Autodesk Fusion 360 part; units mm, degrees
note: some values were not read from the file. Chosen so that the rebuilt part matches the saved one: which bodies a step acts on. Set by a fixed rule: which sketch regions a step uses.
(part 3 of 5)
extrude "Extrude1'''" add sketch "Sketch1 (2)" along normal blind 15 separate body contours L572 L573 L574 L575 picked at (-36.083333, 0.25) makes body 9 in component "grid_3d"
sketch "Sketch2 (3)" plane through (0, 0, -3) normal (0, 0, 1) x (-1, 0, 0) in component "grid_3d"
  line L0 (-108.25, 0.75) -> (-108.25, -0.75)
  line L1 (-108.25, -0.75) -> (108.25, -0.75)
  line L2 (108.25, -0.75) -> (108.25, 0.75)
  line L3 (108.25, 0.75) -> (-108.25, 0.75)
  arc A0 (86, 102) -> (87, 101) centre (87, 102) ccw
  line L4 (87, 101) -> (100.585786, 101)
  arc A1 (100.585786, 101) -> (101.292893, 101.292893) centre (100.585786, 102) ccw
  line L5 (101.292893, 101.292893) -> (116.946699, 116.946699)
  arc A2 (116.946699, 116.946699) -> (122.25, 129.75) centre (122.25, 122.25) ccw
  line L6 (122.25, 129.75) -> (-116.02505, 129.75)
  arc A3 (-116.02505, 129.75) -> (-116.716711, 128.027778) centre (-116.02505, 128.75) ccw
  arc A4 (-115.999634, 117.256712) -> (-116.716711, 128.027778) centre (-122.25, 122.25) ccw
  arc A5 (-115.999634, 117.256712) -> (-115.925445, 115.925445) centre (-115.218338, 116.632551) ccw
  line L7 (-115.925445, 115.925445) -> (-101.292893, 101.292893)
  arc A6 (-101.292893, 101.292893) -> (-100.585786, 101) centre (-100.585786, 102) ccw
  line L8 (-100.585786, 101) -> (-87, 101)
  arc A7 (-87, 101) -> (-86, 102) centre (-87, 102) ccw
  line L9 (-86, 102) -> (-86, 108.5)
  line L10 (-86, 108.5) -> (-84, 108.5)
  line L11 (-84, 108.5) -> (-84, 102)
  arc A8 (-84, 102) -> (-83, 101) centre (-83, 102) ccw
  line L12 (-83, 101) -> (-70, 101)
  arc A9 (-70, 101) -> (-69, 102) centre (-70, 102) ccw
  line L13 (-69, 102) -> (-69, 108.5)
  line L14 (-69, 108.5) -> (-67, 108.5)
  line L15 (-67, 108.5) -> (-67, 102)
  arc A10 (-67, 102) -> (-66, 101) centre (-66, 102) ccw
  line L16 (-66, 101) -> (-53, 101)
  arc A11 (-53, 101) -> (-52, 102) centre (-53, 102) ccw
  line L17 (-52, 102) -> (-52, 108.5)
  line L18 (-52, 108.5) -> (-50, 108.5)
  line L19 (-50, 108.5) -> (-50, 102)
  arc A12 (-50, 102) -> (-49, 101) centre (-49, 102) ccw
  line L20 (-49, 101) -> (-36, 101)
  arc A13 (-36, 101) -> (-35, 102) centre (-36, 102) ccw
  line L21 (-35, 102) -> (-35, 108.5)
  line L22 (-35, 108.5) -> (-33, 108.5)
  line L23 (-33, 108.5) -> (-33, 102)
  arc A14 (-33, 102) -> (-32, 101) centre (-32, 102) ccw
  line L24 (-32, 101) -> (-19, 101)
  arc A15 (-19, 101) -> (-18, 102) centre (-19, 102) ccw
  line L25 (-18, 102) -> (-18, 108.5)
  line L26 (-18, 108.5) -> (-16, 108.5)
  line L27 (-16, 108.5) -> (-16, 102)
  arc A16 (-16, 102) -> (-15, 101) centre (-15, 102) ccw
  line L28 (-15, 101) -> (-2, 101)
  arc A17 (-2, 101) -> (-1, 102) centre (-2, 102) ccw
  line L29 (-1, 102) -> (-1, 108.5)
  line L30 (-1, 108.5) -> (1, 108.5)
  line L31 (1, 108.5) -> (1, 102)
  arc A18 (1, 102) -> (2, 101) centre (2, 102) ccw
  line L32 (2, 101) -> (15, 101)
  arc A19 (15, 101) -> (16, 102) centre (15, 102) ccw
  line L33 (16, 102) -> (16, 108.5)
  line L34 (16, 108.5) -> (18, 108.5)
  line L35 (18, 108.5) -> (18, 102)
  arc A20 (18, 102) -> (19, 101) centre (19, 102) ccw
  line L36 (19, 101) -> (32, 101)
  arc A21 (32, 101) -> (33, 102) centre (32, 102) ccw
  line L37 (33, 102) -> (33, 108.5)
  line L38 (33, 108.5) -> (35, 108.5)
  line L39 (35, 108.5) -> (35, 102)
  arc A22 (35, 102) -> (36, 101) centre (36, 102) ccw
  line L40 (36, 101) -> (49, 101)
  arc A23 (49, 101) -> (50, 102) centre (49, 102) ccw
  line L41 (50, 102) -> (50, 108.5)
  line L42 (50, 108.5) -> (52, 108.5)
  line L43 (52, 108.5) -> (52, 102)
  arc A24 (52, 102) -> (53, 101) centre (53, 102) ccw
  line L44 (53, 101) -> (66, 101)
  arc A25 (66, 101) -> (67, 102) centre (66, 102) ccw
  line L45 (67, 102) -> (67, 108.5)
  line L46 (67, 108.5) -> (69, 108.5)
  line L47 (69, 108.5) -> (69, 102)
  arc A26 (69, 102) -> (70, 101) centre (70, 102) ccw
  line L48 (70, 101) -> (83, 101)
  arc A27 (83, 101) -> (84, 102) centre (83, 102) ccw
  line L49 (84, 102) -> (84, 108.5)
  line L50 (84, 108.5) -> (86, 108.5)
  line L51 (86, 108.5) -> (86, 102)
  circle A28 centre (-17, 118.5) radius 7.5
  circle A29 centre (34, 118.5) radius 7.5
  circle A30 centre (17, 118.5) radius 7.5
  circle A31 centre (122.25, 122.25) radius 2.5
  circle A32 centre (-34, 118.5) radius 7.5
  circle A33 centre (0, 118.5) radius 7.5
  arc A34 (-86, -102) -> (-87, -101) centre (-87, -102) ccw
  line L52 (-87, -101) -> (-100.585786, -101)
  arc A35 (-100.585786, -101) -> (-101.292893, -101.292893) centre (-100.585786, -102) ccw
  line L53 (-101.292893, -101.292893) -> (-116.946699, -116.946699)
  arc A36 (-116.946699, -116.946699) -> (-122.25, -129.75) centre (-122.25, -122.25) ccw
  line L54 (-122.25, -129.75) -> (116.02505, -129.75)
  arc A37 (116.02505, -129.75) -> (116.716711, -128.027778) centre (116.02505, -128.75) ccw
  arc A38 (115.999634, -117.256712) -> (116.716711, -128.027778) centre (122.25, -122.25) ccw
  arc A39 (115.999634, -117.256712) -> (115.925445, -115.925445) centre (115.218338, -116.632551) ccw
  line L55 (115.925445, -115.925445) -> (101.292893, -101.292893)
  arc A40 (101.292893, -101.292893) -> (100.585786, -101) centre (100.585786, -102) ccw
  line L56 (100.585786, -101) -> (87, -101)
  arc A41 (87, -101) -> (86, -102) centre (87, -102) ccw
  line L57 (86, -102) -> (86, -108.5)
  line L58 (86, -108.5) -> (84, -108.5)
  line L59 (84, -108.5) -> (84, -102)
  arc A42 (84, -102) -> (83, -101) centre (83, -102) ccw
  line L60 (83, -101) -> (70, -101)
  arc A43 (70, -101) -> (69, -102) centre (70, -102) ccw
  line L61 (69, -102) -> (69, -108.5)
  line L62 (69, -108.5) -> (67, -108.5)
  line L63 (67, -108.5) -> (67, -102)
  arc A44 (67, -102) -> (66, -101) centre (66, -102) ccw
  line L64 (66, -101) -> (53, -101)
  arc A45 (53, -101) -> (52, -102) centre (53, -102) ccw
  line L65 (52, -102) -> (52, -108.5)
  line L66 (52, -108.5) -> (50, -108.5)
  line L67 (50, -108.5) -> (50, -102)
  arc A46 (50, -102) -> (49, -101) centre (49, -102) ccw
  line L68 (49, -101) -> (36, -101)
  arc A47 (36, -101) -> (35, -102) centre (36, -102) ccw
  line L69 (35, -102) -> (35, -108.5)
  line L70 (35, -108.5) -> (33, -108.5)
  line L71 (33, -108.5) -> (33, -102)
  arc A48 (33, -102) -> (32, -101) centre (32, -102) ccw
  line L72 (32, -101) -> (19, -101)
  arc A49 (19, -101) -> (18, -102) centre (19, -102) ccw
  line L73 (18, -102) -> (18, -108.5)
  line L74 (18, -108.5) -> (16, -108.5)
  line L75 (16, -108.5) -> (16, -102)
  arc A50 (16, -102) -> (15, -101) centre (15, -102) ccw
  line L76 (15, -101) -> (2, -101)
  arc A51 (2, -101) -> (1, -102) centre (2, -102) ccw
  line L77 (1, -102) -> (1, -108.5)
  line L78 (1, -108.5) -> (-1, -108.5)
  line L79 (-1, -108.5) -> (-1, -102)
  arc A52 (-1, -102) -> (-2, -101) centre (-2, -102) ccw
  line L80 (-2, -101) -> (-15, -101)
  arc A53 (-15, -101) -> (-16, -102) centre (-15, -102) ccw
  line L81 (-16, -102) -> (-16, -108.5)
  line L82 (-16, -108.5) -> (-18, -108.5)
  line L83 (-18, -108.5) -> (-18, -102)
  arc A54 (-18, -102) -> (-19, -101) centre (-19, -102) ccw
  line L84 (-19, -101) -> (-32, -101)
  arc A55 (-32, -101) -> (-33, -102) centre (-32, -102) ccw
  line L85 (-33, -102) -> (-33, -108.5)
  line L86 (-33, -108.5) -> (-35, -108.5)
  line L87 (-35, -108.5) -> (-35, -102)
  arc A56 (-35, -102) -> (-36, -101) centre (-36, -102) ccw
  line L88 (-36, -101) -> (-49, -101)
  arc A57 (-49, -101) -> (-50, -102) centre (-49, -102) ccw
  line L89 (-50, -102) -> (-50, -108.5)
  line L90 (-50, -108.5) -> (-52, -108.5)
  line L91 (-52, -108.5) -> (-52, -102)
  arc A58 (-52, -102) -> (-53, -101) centre (-53, -102) ccw
  line L92 (-53, -101) -> (-66, -101)
  arc A59 (-66, -101) -> (-67, -102) centre (-66, -102) ccw
  line L93 (-67, -102) -> (-67, -108.5)
  line L94 (-67, -108.5) -> (-69, -108.5)
  line L95 (-69, -108.5) -> (-69, -102)
  arc A60 (-69, -102) -> (-70, -101) centre (-70, -102) ccw
  line L96 (-70, -101) -> (-83, -101)
  arc A61 (-83, -101) -> (-84, -102) centre (-83, -102) ccw
  line L97 (-84, -102) -> (-84, -108.5)
  line L98 (-84, -108.5) -> (-86, -108.5)
  line L99 (-86, -108.5) -> (-86, -102)
  circle A62 centre (17, -118.5) radius 7.5
  circle A63 centre (-34, -118.5) radius 7.5
  circle A64 centre (-17, -118.5) radius 7.5
  circle A65 centre (-122.25, -122.25) radius 2.5
  circle A66 centre (34, -118.5) radius 7.5
  circle A67 centre (0, -118.5) radius 7.5
  line L100 (1, 129.75) -> (1, -129.75) construction
  line L101 (-1, 129.75) -> (-1, -129.75) construction
  line L102 (-1, 0.75) -> (1, 0.75)
  line L103 (1, 0.75) -> (1, -0.75)
  line L104 (1, -0.75) -> (-1, -0.75)
  line L105 (-1, -0.75) -> (-1, 0.75)
  line L106 (-86, -0.75) -> (-86, 0.75)
  line L107 (-84, 0.75) -> (-84, -0.75)
  line L108 (-69, -0.75) -> (-69, 0.75)
  line L109 (-67, 0.75) -> (-67, -0.75)
  line L110 (-52, -0.75) -> (-52, 0.75)
  line L111 (-50, 0.75) -> (-50, -0.75)
  line L112 (-35, -0.75) -> (-35, 0.75)
  line L113 (-33, 0.75) -> (-33, -0.75)
  line L114 (-18, -0.75) -> (-18, 0.75)
  line L115 (-16, 0.75) -> (-16, -0.75)
  line L116 (16, -0.75) -> (16, 0.75)
  line L117 (18, 0.75) -> (18, -0.75)
  line L118 (33, -0.75) -> (33, 0.75)
  line L119 (35, 0.75) -> (35, -0.75)
  line L120 (50, -0.75) -> (50, 0.75)
  line L121 (52, 0.75) -> (52, -0.75)
  line L122 (67, -0.75) -> (67, 0.75)
  line L123 (69, 0.75) -> (69, -0.75)
  line L124 (84, -0.75) -> (84, 0.75)
  line L125 (86, 0.75) -> (86, -0.75)
  line L126 (-85, 108.5) -> (-85, -108.5) construction
  dimension "d245" = 17
  dimension "d246" = 0
  constraint coincident L6 L100.start
  constraint coincident L54 L100.end
  constraint perpendicular L54 L100
  constraint coincident L6 L101.start
  constraint coincident L54 L101.end
  constraint perpendicular L54 L101
  constraint coincident A51.end L100
  constraint coincident L79.end L101
  constraint horizontal L102
  constraint vertical L103
  constraint horizontal L104
  constraint vertical L105
  constraint coincident L100 L103.end
  constraint coincident L1 L103.end
  constraint coincident L101 L102.start
  constraint coincident L3 L102.start
  constraint midpoint L10 L126.start
  constraint midpoint L98 L126.end
extrude "Extrude2'" cut sketch "Sketch2 (3)" against normal blind 7.75 contours L1 L3 L106 L107 | L1 L3 L108 L109 | L1 L3 L110 L111 | L1 L3 L112 L113 | L1 L3 L114 L115 | L1 L3 L102 L103 L104 L105 | L1 L3 L116 L117 | L1 L3 L118 L119 | L1 L3 L120 L121 | L1 L3 L122 L123 | L1 L3 L124 L125 picked at (-85.333333, 0.25) picked at (-68.333333, 0.25) picked at (-51.333333, 0.25) picked at (-34.333333, -0.25) picked at (-17.333333, -0.25) picked at (-0.333333, -0.25) picked at (16.666667, -0.25) picked at (33.666667, 0.25) picked at (50.666667, 0.25) picked at (67.666667, 0.25) picked at (84.666667, 0.25) bodies 9 in component "grid_3d"
pattern_linear "R-Pattern1" count 11 spacing 17 along (0, 1, 0) both ways of bodies 9 makes body 10 at (-100.833333, -85.75, -10.583333) makes body 11 at (-100.833333, -68.75, -10.583333) makes body 12 at (-100.833333, -51.75, -10.583333) makes body 13 at (-100.833333, -34.75, -10.583333) makes body 14 at (-100.833333, -17.75, -10.583333) makes body 15 at (-100.833333, 16.25, -10.583333) makes body 16 at (-100.833333, 33.25, -10.583333) makes body 17 at (-100.833333, 50.25, -10.583333) makes body 18 at (-100.833333, 67.25, -10.583333) makes body 19 at (-100.833333, 84.25, -10.583333) in component "grid_3d"
copy_body "CopyPasteBodies1" bodies 9 makes body 20 in component "grid_3d"
move_body "Move1" bodies 20 to x (0, 1, 0) y (1, 0, 0) z (0, 0, -1) at (0, 0, -21.5) in component "grid_3d"
extrude "Extrude3''" cut 12 faces at (-0.25, 100.833333, -18.5) (0.25, 79, -18.5) (-0.25, 57, -18.5) (-0.25, 40, -18.5) (-0.25, 28, -18.5) (0.25, 6, -18.5) (-0.25, -6, -18.5) (-0.25, -93.416667, -18.5) (-0.25, -74, -18.5) (-0.25, -57, -18.5) (-0.25, -40, -18.5) (-0.25, -23, -18.5) along direction (0, 0, 1) blind 1 on bodies 20 bodies 20 in component "grid_3d"
pattern_linear "R-Pattern2" count 11 spacing 17 along (1, 0, 0) both ways of bodies 20 makes body 21 at (-84.25, -100.833333, -10.583333) makes body 22 at (-67.25, -100.833333, -10.583333) makes body 23 at (-50.25, -100.833333, -10.583333) makes body 24 at (-33.25, -100.833333, -10.583333) makes body 25 at (-16.25, -100.833333, -10.583333) makes body 26 at (17.75, -100.833333, -10.583333) makes body 27 at (34.75, -100.833333, -10.583333) makes body 28 at (51.75, -100.833333, -10.583333) makes body 29 at (68.75, -100.833333, -10.583333) makes body 30 at (85.75, -100.833333, -10.583333) in component "grid_3d"
sketch "Sketch3 (3)" plane through (0, 0, -21) normal (0, 0, -1) x (1, 0, 0) in component "corner-bracket_3d"
  line L0 (110.5, 70.5) -> (105.75, 70.5)
  line L1 (105.75, 70.5) -> (105.75, 82.5)
  line L2 (105.75, 82.5) -> (110.5, 82.5)
  line L3 (110.5, 82.5) -> (110.5, 70.5)
  circle A0 centre (122.25, 61.125) radius 1.6
  line L4 (110.5, 87.5) -> (105.75, 87.5)
  line L5 (105.75, 87.5) -> (105.75, 99.5)
  line L6 (105.75, 99.5) -> (110.5, 99.5)
  line L7 (110.5, 99.5) -> (110.5, 87.5)
  line L8 (51, -124.5) -> (46.25, -124.5)
  line L9 (46.25, -124.5) -> (46.25, -112.5)
  line L10 (46.25, -112.5) -> (51, -112.5)
  line L11 (51, -112.5) -> (51, -124.5)
  circle A1 centre (0, 118.5) radius 7.5
  circle A2 centre (-61.125, -122.25) radius 1.6
  circle A3 centre (61.125, -122.25) radius 1.6
  circle A4 centre (122.25, -61.125) radius 1.6
  circle A5 centre (-61.125, 122.25) radius 1.6
  circle A6 centre (61.125, 122.25) radius 1.6
  circle A7 centre (-122.25, -61.125) radius 1.6
  circle A8 centre (-122.25, 61.125) radius 1.6
  circle A9 centre (-34, 123) radius 1.6
  circle A10 centre (-17, 123) radius 1.6
  circle A11 centre (17, 123) radius 1.6
  circle A12 centre (34, 123) radius 1.6
  circle A13 centre (-34, 114) radius 1.6
  circle A14 centre (17, 114) radius 1.6
  circle A15 centre (-17, 114) radius 1.6
  circle A16 centre (34, 114) radius 1.6
  circle A17 centre (-122.25, 122.25) radius 2.5
  circle A18 centre (-122.25, -122.25) radius 2.5
  line L12 (-105.75, -2.5) -> (-105.75, -14.5)
  line L13 (-105.75, -14.5) -> (-110.5, -14.5)
  line L14 (-110.5, -14.5) -> (-110.5, -2.5)
  line L15 (-110.5, -2.5) -> (-105.75, -2.5)
  line L16 (-105.75, -87.5) -> (-105.75, -99.5)
  line L17 (-105.75, -99.5) -> (-110.5, -99.5)
  line L18 (-110.5, -99.5) -> (-110.5, -87.5)
  line L19 (-110.5, -87.5) -> (-105.75, -87.5)
  circle A19 centre (122.25, 122.25) radius 2.5
  line L20 (-105.75, -19.5) -> (-105.75, -31.5)
  line L21 (-105.75, -31.5) -> (-110.5, -31.5)
  line L22 (-110.5, -31.5) -> (-110.5, -19.5)
  line L23 (-110.5, -19.5) -> (-105.75, -19.5)
  line L24 (-105.75, -36.5) -> (-105.75, -48.5)
  line L25 (-105.75, -48.5) -> (-110.5, -48.5)
  line L26 (-110.5, -48.5) -> (-110.5, -36.5)
  line L27 (-110.5, -36.5) -> (-105.75, -36.5)
  line L28 (-105.75, -53.5) -> (-105.75, -65.5)
  line L29 (-105.75, -65.5) -> (-110.5, -65.5)
  line L30 (-110.5, -65.5) -> (-110.5, -53.5)
  line L31 (-110.5, -53.5) -> (-105.75, -53.5)
  line L32 (-105.75, -70.5) -> (-105.75, -82.5)
  line L33 (-105.75, -82.5) -> (-110.5, -82.5)
  line L34 (-110.5, -82.5) -> (-110.5, -70.5)
  line L35 (-110.5, -70.5) -> (-105.75, -70.5)
  line L36 (-46.25, -112.5) -> (-46.25, -124.5)
  line L37 (-46.25, -124.5) -> (-51, -124.5)
  line L38 (-51, -124.5) -> (-51, -112.5)
  line L39 (-51, -112.5) -> (-46.25, -112.5)
  line L40 (-105.75, 14.5) -> (-105.75, 2.5)
  line L41 (-105.75, 2.5) -> (-110.5, 2.5)
  line L42 (-110.5, 2.5) -> (-110.5, 14.5)
  line L43 (-110.5, 14.5) -> (-105.75, 14.5)
  line L44 (-105.75, 31.5) -> (-105.75, 19.5)
  line L45 (-105.75, 19.5) -> (-110.5, 19.5)
  line L46 (-110.5, 19.5) -> (-110.5, 31.5)
  line L47 (-110.5, 31.5) -> (-105.75, 31.5)
  line L48 (-105.75, 48.5) -> (-105.75, 36.5)
  line L49 (-105.75, 36.5) -> (-110.5, 36.5)
  line L50 (-110.5, 36.5) -> (-110.5, 48.5)
  line L51 (-110.5, 48.5) -> (-105.75, 48.5)
  line L52 (-105.75, 65.5) -> (-105.75, 53.5)
  line L53 (-105.75, 53.5) -> (-110.5, 53.5)
  line L54 (-110.5, 53.5) -> (-110.5, 65.5)
  line L55 (-110.5, 65.5) -> (-105.75, 65.5)
  line L56 (-105.75, 82.5) -> (-105.75, 70.5)
  line L57 (-105.75, 70.5) -> (-110.5, 70.5)
  line L58 (-110.5, 70.5) -> (-110.5, 82.5)
  line L59 (-110.5, 82.5) -> (-105.75, 82.5)
  line L60 (-105.75, 99.5) -> (-105.75, 87.5)
  line L61 (-105.75, 87.5) -> (-110.5, 87.5)
  line L62 (-110.5, 87.5) -> (-110.5, 99.5)
  line L63 (-110.5, 99.5) -> (-105.75, 99.5)
  line L64 (110.5, -99.5) -> (105.75, -99.5)
  line L65 (105.75, -99.5) -> (105.75, -87.5)
  line L66 (105.75, -87.5) -> (110.5, -87.5)
  line L67 (110.5, -87.5) -> (110.5, -99.5)
  line L68 (110.5, -82.5) -> (105.75, -82.5)
  line L69 (105.75, -82.5) -> (105.75, -70.5)
  line L70 (105.75, -70.5) -> (110.5, -70.5)
  line L71 (110.5, -70.5) -> (110.5, -82.5)
  line L72 (110.5, -65.5) -> (105.75, -65.5)
  line L73 (105.75, -65.5) -> (105.75, -53.5)
  line L74 (105.75, -53.5) -> (110.5, -53.5)
  line L75 (110.5, -53.5) -> (110.5, -65.5)
  line L76 (110.5, -48.5) -> (105.75, -48.5)
  line L77 (105.75, -48.5) -> (105.75, -36.5)
  line L78 (105.75, -36.5) -> (110.5, -36.5)
  line L79 (110.5, -36.5) -> (110.5, -48.5)
  line L80 (110.5, -31.5) -> (105.75, -31.5)
  line L81 (105.75, -31.5) -> (105.75, -19.5)
  line L82 (105.75, -19.5) -> (110.5, -19.5)
  line L83 (110.5, -19.5) -> (110.5, -31.5)
  line L84 (110.5, 36.5) -> (105.75, 36.5)
  line L85 (105.75, 36.5) -> (105.75, 48.5)
  line L86 (105.75, 48.5) -> (110.5, 48.5)
  line L87 (110.5, 48.5) -> (110.5, 36.5)
  line L88 (110.5, -14.5) -> (105.75, -14.5)
  line L89 (105.75, -14.5) -> (105.75, -2.5)
  line L90 (105.75, -2.5) -> (110.5, -2.5)
  line L91 (110.5, -2.5) -> (110.5, -14.5)
  line L92 (110.5, 53.5) -> (105.75, 53.5)
  line L93 (105.75, 53.5) -> (105.75, 65.5)
  line L94 (105.75, 65.5) -> (110.5, 65.5)
  line L95 (110.5, 65.5) -> (110.5, 53.5)
  line L96 (110.5, 2.5) -> (105.75, 2.5)
  line L97 (105.75, 2.5) -> (105.75, 14.5)
  line L98 (105.75, 14.5) -> (110.5, 14.5)
  line L99 (110.5, 14.5) -> (110.5, 2.5)
  line L100 (110.5, 19.5) -> (105.75, 19.5)
  line L101 (105.75, 19.5) -> (105.75, 31.5)
  line L102 (105.75, 31.5) -> (110.5, 31.5)
  line L103 (110.5, 31.5) -> (110.5, 19.5)
  circle A20 centre (122.25, -122.25) radius 2.5
  arc A21 (-129.75, -122.25) -> (-122.25, -129.75) centre (-122.25, -122.25) ccw
  line L104 (-122.25, -129.75) -> (122.25, -129.75)
  arc A22 (122.25, -129.75) -> (129.75, -122.25) centre (122.25, -122.25) ccw
  line L105 (129.75, -122.25) -> (129.75, 122.25)
  arc A23 (129.75, 122.25) -> (122.25, 129.75) centre (122.25, 122.25) ccw
  line L106 (122.25, 129.75) -> (-122.25, 129.75)
  arc A24 (-122.25, 129.75) -> (-129.75, 122.25) centre (-122.25, 122.25) ccw
  line L107 (-129.75, 122.25) -> (-129.75, -122.25)
  circle A25 centre (-122.25, 122.25) radius 2.5
  circle A26 centre (122.25, -122.25) radius 2.5
  circle A27 centre (-122.25, -122.25) radius 2.5
  circle A28 centre (0, -118.5) radius 2.5
  circle A29 centre (122.25, 122.25) radius 2.5
  line L108 (-143.5, 143.5) -> (-143.5, -143.5)
  line L109 (-143.5, -143.5) -> (143.5, -143.5)
  line L110 (143.5, -143.5) -> (143.5, 143.5)
  line L111 (143.5, 143.5) -> (-143.5, 143.5)
  line L112 (-139.5, -139.5) -> (139.5, -139.5)
  line L113 (139.5, -139.5) -> (139.5, 139.5)
  line L114 (139.5, 139.5) -> (-139.5, 139.5)
  line L115 (-139.5, 139.5) -> (-139.5, -139.5)
  circle A30 centre (-122.25, 122.25) radius 7.5 construction
  line L116 (-122.25, 122.25) -> (-139.5, 139.5) construction
  line L117 (-126.822956, 121.02468) -> (-123.47532, 117.677044)
  line L118 (-123.47532, 117.677044) -> (-118.902364, 118.902364)
  line L119 (-118.902364, 118.902364) -> (-117.677044, 123.47532)
  line L120 (-117.677044, 123.47532) -> (-121.02468, 126.822956)
  line L121 (-121.02468, 126.822956) -> (-125.597636, 125.597636)
  line L122 (-125.597636, 125.597636) -> (-126.822956, 121.02468)
  circle A31 centre (-122.25, 122.25) radius 12.5
  line L123 (-121.82233, 139.5) -> (-113.411165, 131.088835)
  line L124 (-139.5, 121.82233) -> (-131.088835, 113.411165)
  line L125 (-129.95, 122.25) -> (-129.95, -122.25)
  line L126 (122.25, 129.95) -> (-122.25, 129.95)
  circle A32 centre (-122.25, 122.25) radius 7.7
  point P0 (-122.25, 122.25)
  dimension "d278" = -4
  dimension "d280" = 4.1
  dimension "d281" = 5
  dimension "d282" = 0.2
  dimension "d283" = 0.2
  dimension "d284" = 0.2
  constraint concentric A25 A30
  constraint coincident L106.end A30
  constraint coincident P0 A17.centre
  constraint parallel L116 L123
  constraint parallel L116 L124
  constraint tangent A31 L124
  constraint tangent A31 L123
  measures "d280" distance of P0 L122
extrude "Extrude4'" add sketch "Sketch3 (3)" along normal blind 25 separate body contours L107 A31 L125 A32 | L106 L107 A31 A32 | L106 A24 L107 A32 | L106 A24 L107 A32 | A31 L125 L126 A32 | L114 L115 A31 L123 L124 | L106 A31 L126 A32 | L117 L118 L119 L120 L121 L122 picked at (-129.853632, 117.997199) picked at (-128.211471, 113.154137) picked at (-123.694175, 129.727794) picked at (-120.88305, 117.129314) picked at (-122.560722, 133.120887) picked at (-129.52366, 137.569009) picked at (-117.997199, 129.853632) picked at (-119.706365, 124.749569) makes body 31 in component "corner-bracket_3d"
extrude "Extrude5'" add sketch "Sketch3 (3)" against normal blind 18 contours A31 L125 L126 A32 | L114 L115 A31 L123 L124 picked at (-122.560722, 133.120887) picked at (-129.52366, 137.569009) bodies 31 in component "corner-bracket_3d"
sketch "Sketch5" plane through (-139.5, 0, 0) normal (-1, 0, 0) x (0, -1, 0) in component "corner-bracket_3d"
  line L0 (121.82233, -3) -> (121.82233, -46)
  line L1 (121.82233, -46) -> (139.5, -46)
  line L2 (139.5, -46) -> (139.5, -3)
  line L3 (139.5, -3) -> (121.82233, -3)
  line L4 (139.5, -20.67767) -> (121.82233, -20.67767) construction
  line L5 (139.5, -20.67767) -> (121.82233, -3) construction
  line L6 (121.82233, -20.67767) -> (139.5, -3) construction
  line L7 (139.5, -24.5) -> (121.82233, -24.5) construction
  circle A0 centre (130.661165, -11.838835) radius 1.75
  circle A1 centre (130.661165, -37.161165) radius 1.75
  dimension "d289" = 17.67767
  dimension "d290" = 17.67767
  dimension "d291" = 3.5
  constraint perpendicular L0 L4
  constraint coincident L2.end L3.start
  constraint coincident L2 L7.start
  constraint perpendicular L0 L7
  constraint midpoint L2 L7.start
  constraint symmetric L7 A0 A1
  measures "d289" distance of L0 L2
  measures "d290" distance of L3 L4
  measures "d291" diameter of A0
extrude "Extrude6" cut sketch "Sketch5" against normal blind 7 contours A0 | A1 picked at (131.451099, -11.382766) picked at (129.871232, -36.705097) bodies 31 in component "corner-bracket_3d"
sketch "Sketch6 (3)" plane through (0, -139.5, 0) normal (0, -1, 0) x (1, 0, 0) in component "corner-bracket_3d"
  line L0 (-139.5, -3) -> (-139.5, -46)
  line L1 (-139.5, -46) -> (-121.82233, -46)
  line L2 (-121.82233, -46) -> (-121.82233, -3)
  line L3 (-121.82233, -3) -> (-139.5, -3)
  line L4 (-139.5, -20.67767) -> (-121.82233, -20.67767) construction
  line L5 (-121.82233, -24.5) -> (-139.5, -24.5) construction
  line L6 (-139.5, -20.67767) -> (-121.82233, -3) construction
  line L7 (-121.82233, -20.67767) -> (-139.5, -3) construction
  circle A0 centre (-130.661165, -11.838835) radius 1.75
  circle A1 centre (-130.661165, -37.161165) radius 1.75
  dimension "d294" = 17.67767
  dimension "d295" = 17.67767
  dimension "d296" = 3.5
  constraint perpendicular L2 L4
  constraint midpoint L0 L5.end
  constraint coincident L0.start L3.end
  constraint symmetric L5 A0 A1
  measures "d295" distance of L3 L4
  measures "d296" diameter of A0
extrude "Extrude7" cut sketch "Sketch6 (3)" against normal blind 7 contours A0 | A1 picked at (-129.871232, -11.382766) picked at (-131.451099, -36.705097) bodies 31 in component "corner-bracket_3d"
sketch "Sketch7 (2)" plane through (0, 0, -46) normal (0, 0, -1) x (1, 0, 0) in component "corner-bracket_3d"
  circle A0 centre (-122.25, 122.25) radius 2.5
  line L0 (-121.82233, 139.5) -> (-139.5, 139.5)
  line L1 (-139.5, 139.5) -> (-139.5, 121.82233)
  line L2 (-139.5, 121.82233) -> (-131.088835, 113.411165)
  arc A1 (-131.088835, 113.411165) -> (-113.411165, 131.088835) centre (-122.25, 122.25) ccw
  line L3 (-113.411165, 131.088835) -> (-121.82233, 139.5)
  line L4 (-125.597636, 125.597636) -> (-126.822956, 121.02468)
  line L5 (-121.02468, 126.822956) -> (-125.597636, 125.597636)
  line L6 (-117.677044, 123.47532) -> (-121.02468, 126.822956)
  line L7 (-118.902364, 118.902364) -> (-117.677044, 123.47532)
  line L8 (-123.47532, 117.677044) -> (-118.902364, 118.902364)
  line L9 (-126.822956, 121.02468) -> (-123.47532, 117.677044)
  line L10 (-132.5, 128.911165) -> (-132.5, 132.411165)
  line L11 (-139.5, 128.911165) -> (-139.5, 132.411165)
  line L12 (-132.411165, 132.5) -> (-128.911165, 132.5)
  line L13 (-132.411165, 139.5) -> (-128.911165, 139.5)
  line L14 (-139.5, 130.661165) -> (-132.5, 130.661165) construction
  line L15 (-125.597636, 125.597636) -> (-139.5, 139.5) construction
  line L16 (-134.5, 133.661165) -> (-137.5, 133.661165)
  line L17 (-137.5, 133.661165) -> (-137.5, 127.661165)
  line L18 (-137.5, 127.661165) -> (-134.5, 127.661165)
  line L19 (-134.5, 127.661165) -> (-134.5, 133.661165)
  line L20 (-134.5, 133.661165) -> (-137.5, 127.661165) construction
  line L21 (-137.5, 133.661165) -> (-134.5, 127.661165) construction
  line L22 (-133.661165, 134.5) -> (-133.661165, 137.5)
  line L23 (-133.661165, 137.5) -> (-127.661165, 137.5)
  line L24 (-127.661165, 137.5) -> (-127.661165, 134.5)
  line L25 (-127.661165, 134.5) -> (-133.661165, 134.5)
  circle A2 centre (-129.840277, 129.840277) radius 1.6
  line L26 (-127.390787, 127.390787) -> (-126.494211, 130.736852)
  line L27 (-126.494211, 130.736852) -> (-128.943701, 133.186342)
  line L28 (-128.943701, 133.186342) -> (-132.289766, 132.289766)
  line L29 (-132.289766, 132.289766) -> (-133.186342, 128.943701)
  line L30 (-133.186342, 128.943701) -> (-130.736852, 126.494211)
  line L31 (-130.736852, 126.494211) -> (-127.390787, 127.390787)
  point P0 (-136, 130.661165)
  point P1 (-129.840277, 129.840277)
  dimension "d301" = 3
  dimension "d302" = 6
  dimension "d305" = 2
  dimension "d309" = 3.2
  dimension "d311" = 6
  dimension "d312" = 3
  constraint coincident L0.end L1.start
  constraint horizontal L16
  constraint perpendicular L16 L17
  constraint parallel L16 L18
  constraint parallel L17 L19
  measures "d302" distance of L16 L18
  measures "d309" diameter of A2
extrude "Extrude8" cut sketch "Sketch7 (2)" against normal blind 21 contours L4 L5 L6 L7 L8 L9 picked at (-125.686508, 123.203068) bodies 31 in component "corner-bracket_3d"
extrude "Extrude9" cut sketch "Sketch7 (2)" against normal blind 37.642 contours L16 L17 L18 L19 | L22 L23 L24 L25 picked at (-135.5, 129.661165) picked at (-129.661165, 135.5) bodies 31 in component "corner-bracket_3d"
extrude "Extrude10" cut sketch "Sketch7 (2)" against normal blind 3 contours A2 picked at (-129.449316, 130.362014) bodies 31 in component "corner-bracket_3d"
sketch "Sketch9" plane through (0, 0, -43) normal (0, 0, -1) x (1, 0, 0) in component "corner-bracket_3d"
  circle A0 centre (-129.840277, 129.840277) radius 1.6
  line L0 (-132.289766, 132.289766) -> (-133.186342, 128.943701)
  line L1 (-128.943701, 133.186342) -> (-132.289766, 132.289766)
  line L2 (-126.494211, 130.736852) -> (-128.943701, 133.186342)
  line L3 (-127.390787, 127.390787) -> (-126.494211, 130.736852)
  line L4 (-130.736852, 126.494211) -> (-127.390787, 127.390787)
  line L5 (-133.186342, 128.943701) -> (-130.736852, 126.494211)
extrude "Extrude11" cut sketch "Sketch9" against normal blind 3 bodies 31 in component "corner-bracket_3d"
extrude "Extrude12" cut sketch "Sketch9" against normal blind 10 contours A0 picked at (-129.3129, 129.194248) bodies 31 in component "corner-bracket_3d"
fillet "Fillet2'" radius 1 3 edges at (-139.5, -139.5, -24.5) (-139.5, -121.82233, -24.5) (-121.82233, -139.5, -24.5) on bodies 31 in component "corner-bracket_3d"
fillet "Fillet3" radius 1 2 edges at (-129.95, -112.403173, -12) (-112.403173, -129.95, -12) on bodies 31 in component "corner-bracket_3d"
pattern_circular "C-Pattern1'" count 4 over 360 about axis through (0, 0, 1.75) along (0, 0, 1) of bodies 31 makes body 32 at (114.578815, -112.380708, -37.666667) makes body 33 at (110.671913, 126.961465, -29.333333) makes body 34 at (-112.010599, 115.080295, -37.666667) in component "corner-bracket_3d"
sketch "Sketch1 (3)" plane through (0, 0, -18) normal (0, 0, 1) x (-1, 0, 0) in component "edge-bracket_3d"
  line L0 (-105.75, 70.5) -> (-110.5, 70.5)
  line L1 (-110.5, 70.5) -> (-110.5, 82.5)
  line L2 (-110.5, 82.5) -> (-105.75, 82.5)
  line L3 (-105.75, 82.5) -> (-105.75, 70.5)
  circle A0 centre (-122.25, 61.125) radius 1.6
  line L4 (-105.75, 87.5) -> (-110.5, 87.5)
  line L5 (-110.5, 87.5) -> (-110.5, 99.5)
  line L6 (-110.5, 99.5) -> (-105.75, 99.5)
  line L7 (-105.75, 99.5) -> (-105.75, 87.5)
  line L8 (-46.25, -124.5) -> (-51, -124.5)
  line L9 (-51, -124.5) -> (-51, -112.5)
  line L10 (-51, -112.5) -> (-46.25, -112.5)
  line L11 (-46.25, -112.5) -> (-46.25, -124.5)
  circle A1 centre (0, 118.5) radius 7.5
  circle A2 centre (61.125, -122.25) radius 1.6
  circle A3 centre (-61.125, -122.25) radius 1.6
  circle A4 centre (-122.25, -61.125) radius 1.6
  circle A5 centre (61.125, 122.25) radius 1.6
  circle A6 centre (-61.125, 122.25) radius 1.6
  circle A7 centre (122.25, -61.125) radius 1.6
  circle A8 centre (122.25, 61.125) radius 1.6
  circle A9 centre (34, 123) radius 1.6
  circle A10 centre (17, 123) radius 1.6
  circle A11 centre (-17, 123) radius 1.6
  circle A12 centre (-34, 123) radius 1.6
  circle A13 centre (34, 114) radius 1.6
  circle A14 centre (-17, 114) radius 1.6
  circle A15 centre (17, 114) radius 1.6
  circle A16 centre (-34, 114) radius 1.6
  circle A17 centre (122.25, 122.25) radius 2.5
  circle A18 centre (122.25, -122.25) radius 2.5
  line L12 (105.75, -14.5) -> (105.75, -2.5)
  line L13 (105.75, -2.5) -> (110.5, -2.5)
  line L14 (110.5, -2.5) -> (110.5, -14.5)
  line L15 (110.5, -14.5) -> (105.75, -14.5)
  line L16 (105.75, -99.5) -> (105.75, -87.5)
  line L17 (105.75, -87.5) -> (110.5, -87.5)
  line L18 (110.5, -87.5) -> (110.5, -99.5)
  line L19 (110.5, -99.5) -> (105.75, -99.5)
  circle A19 centre (-122.25, 122.25) radius 2.5
  line L20 (105.75, -31.5) -> (105.75, -19.5)
  line L21 (105.75, -19.5) -> (110.5, -19.5)
  line L22 (110.5, -19.5) -> (110.5, -31.5)
  line L23 (110.5, -31.5) -> (105.75, -31.5)
  line L24 (105.75, -48.5) -> (105.75, -36.5)
  line L25 (105.75, -36.5) -> (110.5, -36.5)
  line L26 (110.5, -36.5) -> (110.5, -48.5)
  line L27 (110.5, -48.5) -> (105.75, -48.5)
  line L28 (105.75, -65.5) -> (105.75, -53.5)
  line L29 (105.75, -53.5) -> (110.5, -53.5)
  line L30 (110.5, -53.5) -> (110.5, -65.5)
  line L31 (110.5, -65.5) -> (105.75, -65.5)
  line L32 (105.75, -82.5) -> (105.75, -70.5)
  line L33 (105.75, -70.5) -> (110.5, -70.5)
  line L34 (110.5, -70.5) -> (110.5, -82.5)
  line L35 (110.5, -82.5) -> (105.75, -82.5)
  line L36 (46.25, -124.5) -> (46.25, -112.5)
  line L37 (46.25, -112.5) -> (51, -112.5)
  line L38 (51, -112.5) -> (51, -124.5)
  line L39 (51, -124.5) -> (46.25, -124.5)
  line L40 (105.75, 2.5) -> (105.75, 14.5)
  line L41 (105.75, 14.5) -> (110.5, 14.5)
  line L42 (110.5, 14.5) -> (110.5, 2.5)
  line L43 (110.5, 2.5) -> (105.75, 2.5)
  line L44 (105.75, 19.5) -> (105.75, 31.5)
  line L45 (105.75, 31.5) -> (110.5, 31.5)
  line L46 (110.5, 31.5) -> (110.5, 19.5)
  line L47 (110.5, 19.5) -> (105.75, 19.5)
  line L48 (105.75, 36.5) -> (105.75, 48.5)
  line L49 (105.75, 48.5) -> (110.5, 48.5)
  line L50 (110.5, 48.5) -> (110.5, 36.5)
  line L51 (110.5, 36.5) -> (105.75, 36.5)
  line L52 (105.75, 53.5) -> (105.75, 65.5)
  line L53 (105.75, 65.5) -> (110.5, 65.5)
  line L54 (110.5, 65.5) -> (110.5, 53.5)
  line L55 (110.5, 53.5) -> (105.75, 53.5)
  line L56 (105.75, 70.5) -> (105.75, 82.5)
  line L57 (105.75, 82.5) -> (110.5, 82.5)
  line L58 (110.5, 82.5) -> (110.5, 70.5)
  line L59 (110.5, 70.5) -> (105.75, 70.5)
  line L60 (105.75, 87.5) -> (105.75, 99.5)
  line L61 (105.75, 99.5) -> (110.5, 99.5)
  line L62 (110.5, 99.5) -> (110.5, 87.5)
  line L63 (110.5, 87.5) -> (105.75, 87.5)
  line L64 (-105.75, -99.5) -> (-110.5, -99.5)
  line L65 (-110.5, -99.5) -> (-110.5, -87.5)
  line L66 (-110.5, -87.5) -> (-105.75, -87.5)
  line L67 (-105.75, -87.5) -> (-105.75, -99.5)
  line L68 (-105.75, -82.5) -> (-110.5, -82.5)
  line L69 (-110.5, -82.5) -> (-110.5, -70.5)
  line L70 (-110.5, -70.5) -> (-105.75, -70.5)
  line L71 (-105.75, -70.5) -> (-105.75, -82.5)
  line L72 (-105.75, -65.5) -> (-110.5, -65.5)
  line L73 (-110.5, -65.5) -> (-110.5, -53.5)
  line L74 (-110.5, -53.5) -> (-105.75, -53.5)
  line L75 (-105.75, -53.5) -> (-105.75, -65.5)
  line L76 (-105.75, -48.5) -> (-110.5, -48.5)
  line L77 (-110.5, -48.5) -> (-110.5, -36.5)
  line L78 (-110.5, -36.5) -> (-105.75, -36.5)
  line L79 (-105.75, -36.5) -> (-105.75, -48.5)
  line L80 (-105.75, -31.5) -> (-110.5, -31.5)
  line L81 (-110.5, -31.5) -> (-110.5, -19.5)
  line L82 (-110.5, -19.5) -> (-105.75, -19.5)
  line L83 (-105.75, -19.5) -> (-105.75, -31.5)
  line L84 (-105.75, 36.5) -> (-110.5, 36.5)
  line L85 (-110.5, 36.5) -> (-110.5, 48.5)
  line L86 (-110.5, 48.5) -> (-105.75, 48.5)
  line L87 (-105.75, 48.5) -> (-105.75, 36.5)
  line L88 (-105.75, -14.5) -> (-110.5, -14.5)
  line L89 (-110.5, -14.5) -> (-110.5, -2.5)
  line L90 (-110.5, -2.5) -> (-105.75, -2.5)
  line L91 (-105.75, -2.5) -> (-105.75, -14.5)
  line L92 (-105.75, 53.5) -> (-110.5, 53.5)
  line L93 (-110.5, 53.5) -> (-110.5, 65.5)
  line L94 (-110.5, 65.5) -> (-105.75, 65.5)
  line L95 (-105.75, 65.5) -> (-105.75, 53.5)
  line L96 (-105.75, 2.5) -> (-110.5, 2.5)
  line L97 (-110.5, 2.5) -> (-110.5, 14.5)
  line L98 (-110.5, 14.5) -> (-105.75, 14.5)
  line L99 (-105.75, 14.5) -> (-105.75, 2.5)
  line L100 (-105.75, 19.5) -> (-110.5, 19.5)
  line L101 (-110.5, 19.5) -> (-110.5, 31.5)
  line L102 (-110.5, 31.5) -> (-105.75, 31.5)
  line L103 (-105.75, 31.5) -> (-105.75, 19.5)
  circle A20 centre (-122.25, -122.25) radius 2.5
  arc A21 (122.25, -129.75) -> (129.75, -122.25) centre (122.25, -122.25) ccw
  line L104 (129.75, -122.25) -> (129.75, 122.25)
  arc A22 (129.75, 122.25) -> (122.25, 129.75) centre (122.25, 122.25) ccw
  line L105 (122.25, 129.75) -> (-122.25, 129.75)
  arc A23 (-122.25, 129.75) -> (-129.75, 122.25) centre (-122.25, 122.25) ccw
  line L106 (-129.75, 122.25) -> (-129.75, -122.25)
  arc A24 (-129.75, -122.25) -> (-122.25, -129.75) centre (-122.25, -122.25) ccw
  line L107 (-122.25, -129.75) -> (122.25, -129.75)
  line L108 (68.625, 128.75) -> (68.625, 122.25)
  arc A25 (53.625, 122.25) -> (68.625, 122.25) centre (61.125, 122.25) ccw
  line L109 (53.625, 122.25) -> (53.625, 128.75)
  arc A26 (53.625, 128.75) -> (52.625, 129.75) centre (52.625, 128.75) ccw
  line L110 (52.625, 129.75) -> (69.625, 129.75)
  arc A27 (69.625, 129.75) -> (68.625, 128.75) centre (69.625, 128.75) ccw
  arc A28 (122.236544, 139.5) -> (121.529437, 139.207107) centre (122.236544, 138.5) ccw
  line L111 (122.236544, 139.5) -> (138.5, 139.5)
  arc A29 (139.5, 138.5) -> (138.5, 139.5) centre (138.5, 138.5) ccw
  line L112 (139.5, 138.5) -> (139.5, 122.236544)
  arc A30 (139.207107, 121.529437) -> (139.5, 122.236544) centre (138.5, 122.236544) ccw
  line L113 (139.207107, 121.529437) -> (131.088835, 113.411165)
  arc A31 (113.411165, 131.088835) -> (131.088835, 113.411165) centre (122.25, 122.25) ccw
  line L114 (113.411165, 131.088835) -> (121.529437, 139.207107)
  circle A32 centre (129.840277, 129.840277) radius 1.6
  line L115 (137.5, 133.661165) -> (134.5, 133.661165)
  line L116 (134.5, 133.661165) -> (134.5, 127.661165)
  line L117 (134.5, 127.661165) -> (137.5, 127.661165)
  line L118 (137.5, 127.661165) -> (137.5, 133.661165)
  line L119 (133.661165, 137.5) -> (127.661165, 137.5)
  line L120 (127.661165, 137.5) -> (127.661165, 134.5)
  line L121 (127.661165, 134.5) -> (133.661165, 134.5)
  line L122 (133.661165, 134.5) -> (133.661165, 137.5)
  line L123 (118.902364, 118.902364) -> (123.47532, 117.677044)
  line L124 (123.47532, 117.677044) -> (126.822956, 121.02468)
  line L125 (126.822956, 121.02468) -> (125.597636, 125.597636)
  line L126 (125.597636, 125.597636) -> (121.02468, 126.822956)
  line L127 (121.02468, 126.822956) -> (117.677044, 123.47532)
  line L128 (117.677044, 123.47532) -> (118.902364, 118.902364)
  line L129 (59.392949, 125.25) -> (57.660898, 122.25)
  line L130 (57.660898, 122.25) -> (59.392949, 119.25)
  line L131 (59.392949, 119.25) -> (62.857051, 119.25)
  line L132 (62.857051, 119.25) -> (64.589102, 122.25)
  line L133 (64.589102, 122.25) -> (62.857051, 125.25)
  line L134 (62.857051, 125.25) -> (59.392949, 125.25)
  line L135 (68.425, 128.75) -> (68.425, 122.25)
  arc A33 (53.825, 122.25) -> (68.425, 122.25) centre (61.125, 122.25) ccw
  line L136 (53.825, 122.25) -> (53.825, 128.75)
  arc A34 (53.825, 128.75) -> (53.519427, 129.55) centre (52.625, 128.75) ccw
  line L137 (53.519427, 129.55) -> (68.730573, 129.55) construction
  arc A35 (68.730573, 129.55) -> (68.425, 128.75) centre (69.625, 128.75) ccw
  line L138 (53.825, 128.75) -> (53.825, 139.5)
  line L139 (53.825, 139.5) -> (68.425, 139.5)
  line L140 (68.425, 139.5) -> (68.425, 128.75)
  point P0 (61.125, 122.25)
  dimension "d325" = 3
  dimension "d326" = -0.2
  constraint coincident P0 A5.centre
  constraint horizontal L134
  constraint tangent A34 L138
  constraint perpendicular L110 L138
  constraint perpendicular L138 L139
  constraint perpendicular L139 L140
  measures "d325" distance of P0 L134
extrude "Extrude1''''" add sketch "Sketch1 (3)" along normal blind 2.5 separate body contours L105 L110 L135 A33 L136 L138 L140 | L105 L110 L138 L139 L140 | L129 L130 L131 L132 L133 L134 picked at (61.70235, 128.25) picked at (63.558333, 133) picked at (61.085144, 119.718158) makes body 35 in component "edge-bracket_3d"
sketch "Sketch2 (4)" plane through (0, 0, -15.5) normal (0, 0, 1) x (-1, 0, 0) in component "edge-bracket_3d"
  circle A0 centre (61.125, 122.25) radius 1.6
  arc A1 (53.825, 122.25) -> (68.425, 122.25) centre (61.125, 122.25) ccw
  line L0 (68.425, 122.25) -> (68.425, 139.5)
  line L1 (68.425, 139.5) -> (53.825, 139.5)
  line L2 (53.825, 139.5) -> (53.825, 122.25)
  line L3 (64.589102, 122.25) -> (62.857051, 125.25)
  line L4 (62.857051, 125.25) -> (59.392949, 125.25)
  line L5 (59.392949, 125.25) -> (57.660898, 122.25)
  line L6 (57.660898, 122.25) -> (59.392949, 119.25)
  line L7 (59.392949, 119.25) -> (62.857051, 119.25)
  line L8 (62.857051, 119.25) -> (64.589102, 122.25)
extrude "Extrude2''" add sketch "Sketch2 (4)" along normal blind 8 contours A1 L0 L1 L2 picked at (60.54765, 134.75) bodies 35 in component "edge-bracket_3d"
sketch "Sketch3 (4)" plane through (0, 0, -7.5) normal (0, 0, 1) x (-1, 0, 0) in component "edge-bracket_3d"
  line L0 (64.589102, 122.25) -> (62.857051, 119.25)
  line L1 (62.857051, 119.25) -> (59.392949, 119.25)
  line L2 (59.392949, 119.25) -> (57.660898, 122.25)
  line L3 (57.660898, 122.25) -> (59.392949, 125.25)
  line L4 (59.392949, 125.25) -> (62.857051, 125.25)
  line L5 (62.857051, 125.25) -> (64.589102, 122.25)
  line L6 (53.825, 139.5) -> (53.825, 122.25)
  arc A0 (53.825, 122.25) -> (68.425, 122.25) centre (61.125, 122.25) ccw
  line L7 (68.425, 122.25) -> (68.425, 139.5)
  line L8 (68.425, 139.5) -> (53.825, 139.5)
  line L9 (122.25, 129.75) -> (-116.02505, 129.75)
  line L10 (122.25, 130.25) -> (-116.02505, 130.25)
  dimension "d331" = 0.5
extrude "Extrude3'''" add sketch "Sketch3 (4)" along normal blind 4.5 and the other way blind 38.5 contours L6 L7 L8 L10 picked at (63.558333, 136.416667) bodies 35 in component "edge-bracket_3d"
sketch "Sketch4 (2)" plane through (0, 0, -21) normal (0, 0, -1) x (1, 0, 0) in component "edge-bracket_3d"
  line L0 (110.5, 70.5) -> (105.75, 70.5)
  line L1 (105.75, 70.5) -> (105.75, 82.5)
  line L2 (105.75, 82.5) -> (110.5, 82.5)
  line L3 (110.5, 82.5) -> (110.5, 70.5)
  circle A0 centre (122.25, 61.125) radius 1.6
  line L4 (110.5, 87.5) -> (105.75, 87.5)
  line L5 (105.75, 87.5) -> (105.75, 99.5)
  line L6 (105.75, 99.5) -> (110.5, 99.5)
  line L7 (110.5, 99.5) -> (110.5, 87.5)
  line L8 (51, -124.5) -> (46.25, -124.5)
  line L9 (46.25, -124.5) -> (46.25, -112.5)
  line L10 (46.25, -112.5) -> (51, -112.5)
  line L11 (51, -112.5) -> (51, -124.5)
  circle A1 centre (0, 118.5) radius 7.5
  circle A2 centre (-61.125, -122.25) radius 1.6
  circle A3 centre (61.125, -122.25) radius 1.6
  circle A4 centre (122.25, -61.125) radius 1.6
  circle A5 centre (-61.125, 122.25) radius 1.6
  circle A6 centre (61.125, 122.25) radius 1.6
  circle A7 centre (-122.25, -61.125) radius 1.6
  circle A8 centre (-122.25, 61.125) radius 1.6
  circle A9 centre (-34, 123) radius 1.6
  circle A10 centre (-17, 123) radius 1.6
  circle A11 centre (17, 123) radius 1.6
  circle A12 centre (34, 123) radius 1.6
  circle A13 centre (-34, 114) radius 1.6
  circle A14 centre (17, 114) radius 1.6
  circle A15 centre (-17, 114) radius 1.6
  circle A16 centre (34, 114) radius 1.6
  circle A17 centre (-122.25, 122.25) radius 2.5
  circle A18 centre (-122.25, -122.25) radius 2.5
  line L12 (-105.75, -2.5) -> (-105.75, -14.5)
  line L13 (-105.75, -14.5) -> (-110.5, -14.5)
  line L14 (-110.5, -14.5) -> (-110.5, -2.5)
  line L15 (-110.5, -2.5) -> (-105.75, -2.5)
  line L16 (-105.75, -87.5) -> (-105.75, -99.5)
  line L17 (-105.75, -99.5) -> (-110.5, -99.5)
  line L18 (-110.5, -99.5) -> (-110.5, -87.5)
  line L19 (-110.5, -87.5) -> (-105.75, -87.5)
  circle A19 centre (122.25, 122.25) radius 2.5
  line L20 (-105.75, -19.5) -> (-105.75, -31.5)
  line L21 (-105.75, -31.5) -> (-110.5, -31.5)
  line L22 (-110.5, -31.5) -> (-110.5, -19.5)
  line L23 (-110.5, -19.5) -> (-105.75, -19.5)
  line L24 (-105.75, -36.5) -> (-105.75, -48.5)
  line L25 (-105.75, -48.5) -> (-110.5, -48.5)
  line L26 (-110.5, -48.5) -> (-110.5, -36.5)
  line L27 (-110.5, -36.5) -> (-105.75, -36.5)
  line L28 (-105.75, -53.5) -> (-105.75, -65.5)
  line L29 (-105.75, -65.5) -> (-110.5, -65.5)
  line L30 (-110.5, -65.5) -> (-110.5, -53.5)
  line L31 (-110.5, -53.5) -> (-105.75, -53.5)
  line L32 (-105.75, -70.5) -> (-105.75, -82.5)
  line L33 (-105.75, -82.5) -> (-110.5, -82.5)
  line L34 (-110.5, -82.5) -> (-110.5, -70.5)
  line L35 (-110.5, -70.5) -> (-105.75, -70.5)
  line L36 (-46.25, -112.5) -> (-46.25, -124.5)
  line L37 (-46.25, -124.5) -> (-51, -124.5)
  line L38 (-51, -124.5) -> (-51, -112.5)
  line L39 (-51, -112.5) -> (-46.25, -112.5)
  line L40 (-105.75, 14.5) -> (-105.75, 2.5)
  line L41 (-105.75, 2.5) -> (-110.5, 2.5)
  line L42 (-110.5, 2.5) -> (-110.5, 14.5)
  line L43 (-110.5, 14.5) -> (-105.75, 14.5)
  line L44 (-105.75, 31.5) -> (-105.75, 19.5)
  line L45 (-105.75, 19.5) -> (-110.5, 19.5)
  line L46 (-110.5, 19.5) -> (-110.5, 31.5)
  line L47 (-110.5, 31.5) -> (-105.75, 31.5)
  line L48 (-105.75, 48.5) -> (-105.75, 36.5)
  line L49 (-105.75, 36.5) -> (-110.5, 36.5)
  line L50 (-110.5, 36.5) -> (-110.5, 48.5)
  line L51 (-110.5, 48.5) -> (-105.75, 48.5)
  line L52 (-105.75, 65.5) -> (-105.75, 53.5)
  line L53 (-105.75, 53.5) -> (-110.5, 53.5)
  line L54 (-110.5, 53.5) -> (-110.5, 65.5)
  line L55 (-110.5, 65.5) -> (-105.75, 65.5)
  line L56 (-105.75, 82.5) -> (-105.75, 70.5)
  line L57 (-105.75, 70.5) -> (-110.5, 70.5)
  line L58 (-110.5, 70.5) -> (-110.5, 82.5)
  line L59 (-110.5, 82.5) -> (-105.75, 82.5)
  line L60 (-105.75, 99.5) -> (-105.75, 87.5)
  line L61 (-105.75, 87.5) -> (-110.5, 87.5)
  line L62 (-110.5, 87.5) -> (-110.5, 99.5)
  line L63 (-110.5, 99.5) -> (-105.75, 99.5)
  line L64 (110.5, -99.5) -> (105.75, -99.5)
  line L65 (105.75, -99.5) -> (105.75, -87.5)
  line L66 (105.75, -87.5) -> (110.5, -87.5)
  line L67 (110.5, -87.5) -> (110.5, -99.5)
  line L68 (110.5, -82.5) -> (105.75, -82.5)
  line L69 (105.75, -82.5) -> (105.75, -70.5)
  line L70 (105.75, -70.5) -> (110.5, -70.5)
  line L71 (110.5, -70.5) -> (110.5, -82.5)
  line L72 (110.5, -65.5) -> (105.75, -65.5)
  line L73 (105.75, -65.5) -> (105.75, -53.5)
  line L74 (105.75, -53.5) -> (110.5, -53.5)
  line L75 (110.5, -53.5) -> (110.5, -65.5)
  line L76 (110.5, -48.5) -> (105.75, -48.5)
  line L77 (105.75, -48.5) -> (105.75, -36.5)
  line L78 (105.75, -36.5) -> (110.5, -36.5)
  line L79 (110.5, -36.5) -> (110.5, -48.5)
  line L80 (110.5, -31.5) -> (105.75, -31.5)
  line L81 (105.75, -31.5) -> (105.75, -19.5)
  line L82 (105.75, -19.5) -> (110.5, -19.5)
  line L83 (110.5, -19.5) -> (110.5, -31.5)
  line L84 (110.5, 36.5) -> (105.75, 36.5)
  line L85 (105.75, 36.5) -> (105.75, 48.5)
  line L86 (105.75, 48.5) -> (110.5, 48.5)
  line L87 (110.5, 48.5) -> (110.5, 36.5)
  line L88 (110.5, -14.5) -> (105.75, -14.5)
  line L89 (105.75, -14.5) -> (105.75, -2.5)
  line L90 (105.75, -2.5) -> (110.5, -2.5)
  line L91 (110.5, -2.5) -> (110.5, -14.5)
  line L92 (110.5, 53.5) -> (105.75, 53.5)
  line L93 (105.75, 53.5) -> (105.75, 65.5)
  line L94 (105.75, 65.5) -> (110.5, 65.5)
  line L95 (110.5, 65.5) -> (110.5, 53.5)
  line L96 (110.5, 2.5) -> (105.75, 2.5)
  line L97 (105.75, 2.5) -> (105.75, 14.5)
  line L98 (105.75, 14.5) -> (110.5, 14.5)
  line L99 (110.5, 14.5) -> (110.5, 2.5)
  line L100 (110.5, 19.5) -> (105.75, 19.5)
  line L101 (105.75, 19.5) -> (105.75, 31.5)
  line L102 (105.75, 31.5) -> (110.5, 31.5)
  line L103 (110.5, 31.5) -> (110.5, 19.5)
  circle A20 centre (122.25, -122.25) radius 2.5
  arc A21 (-129.75, -122.25) -> (-122.25, -129.75) centre (-122.25, -122.25) ccw
  line L104 (-122.25, -129.75) -> (122.25, -129.75)
  arc A22 (122.25, -129.75) -> (129.75, -122.25) centre (122.25, -122.25) ccw
  line L105 (129.75, -122.25) -> (129.75, 122.25)
  arc A23 (129.75, 122.25) -> (122.25, 129.75) centre (122.25, 122.25) ccw
  line L106 (122.25, 129.75) -> (-122.25, 129.75)
  arc A24 (-122.25, 129.75) -> (-129.75, 122.25) centre (-122.25, 122.25) ccw
  line L107 (-129.75, 122.25) -> (-129.75, -122.25)
  line L108 (-53.825, 130.25) -> (-68.425, 130.25)
  line L109 (-68.425, 130.25) -> (-68.425, 122.25)
  arc A25 (-68.425, 122.25) -> (-53.825, 122.25) centre (-61.125, 122.25) ccw
  line L110 (-53.825, 122.25) -> (-53.825, 130.25)
  circle A26 centre (-61.125, 122.25) radius 1.6
extrude "Extrude4''" add sketch "Sketch4 (2)" along normal blind 2.5 contours L106 L108 L109 L110 | L106 L109 A25 L110 picked at (-63.558333, 129.916667) picked at (-61.164856, 127.781842) bodies 35 in component "edge-bracket_3d"
sketch "Sketch5 (2)" plane through (0, -139.5, 0) normal (0, -1, 0) x (1, 0, 0) in component "edge-bracket_3d"
  line L0 (-53.825, -46) -> (-53.825, -3)
  line L1 (-53.825, -3) -> (-68.425, -3)
  line L2 (-68.425, -3) -> (-68.425, -46)
  line L3 (-68.425, -46) -> (-53.825, -46)
  circle A0 centre (-130.661165, -37.161165) radius 1.75
  circle A1 centre (-130.661165, -37.161165) radius 1.75
  circle A2 centre (-130.661165, -11.838835) radius 1.75
  line L4 (-122.236544, -46) -> (-122.236544, -3)
  line L5 (-122.236544, -3) -> (-138.5, -3)
  line L6 (-138.5, -3) -> (-138.5, -46)
  line L7 (-138.5, -46) -> (-122.236544, -46)
  line L8 (-61.125, -46) -> (-61.125, -3) construction
  circle A3 centre (-61.125, -11.838835) radius 1.6
  circle A4 centre (-61.125, -37.161165) radius 1.6
  dimension "d338" = 3.2
  constraint midpoint L3 L8.start
  constraint midpoint L1 L8.end
  constraint equal A3 A4
  measures "d338" diameter of A3
extrude "Extrude5''" cut sketch "Sketch5 (2)" against normal blind 7 contours A3 | A4 picked at (-60.858333, -11.062549) picked at (-60.858333, -36.38488) bodies 35 in component "edge-bracket_3d"
sketch "Sketch6 (4)" plane through (0, -132.5, 0) normal (0, -1, 0) x (1, 0, 0) in component "edge-bracket_3d"
  circle A0 centre (-61.125, -11.838835) radius 1.6
  line L0 (-61.125, -11.838835) -> (-61.125, -13.438835)
  line L1 (-61.125, -15.418406) -> (-58.025, -13.628621)
  line L2 (-58.025, -13.628621) -> (-58.025, -10.049049)
  line L3 (-58.025, -10.049049) -> (-61.125, -8.259263)
  line L4 (-61.125, -8.259263) -> (-64.225, -10.049049)
  line L5 (-64.225, -10.049049) -> (-64.225, -13.628621)
  line L6 (-64.225, -13.628621) -> (-61.125, -15.418406)
  line L7 (-121.82233, -24.5) -> (-139.5, -24.5)
  line L8 (-61.125, -33.581594) -> (-58.025, -35.371379)
  line L9 (-64.225, -35.371379) -> (-61.125, -33.581594)
  line L10 (-64.225, -38.950951) -> (-64.225, -35.371379)
  line L11 (-61.125, -40.740737) -> (-64.225, -38.950951)
  line L12 (-58.025, -38.950951) -> (-61.125, -40.740737)
  line L13 (-58.025, -35.371379) -> (-58.025, -38.950951)
  point P0 (-61.125, -11.838835)
  dimension "d341" = 3.1
  constraint vertical L0
extrude "Extrude6'" cut sketch "Sketch6 (4)" along normal blind 3 contours A0 | L1 L2 L3 L4 L5 L6 | L8 L9 L10 L11 L12 L13 picked at (-61.099459, -11.331733) picked at (-62.454637, -14.072071) picked at (-61.125, -35.967975) bodies 35 in component "edge-bracket_3d"
extrude "Extrude7'" cut sketch "Sketch5 (2)" against normal blind 10 contours A3 | A4 picked at (-60.858333, -11.062549) picked at (-60.858333, -36.38488) bodies 35 in component "edge-bracket_3d"
fillet "Fillet1'" radius 1 6 edges at (-68.425, -139.5, -24.5) (-53.825, -139.5, -24.5) (-68.425, -130.25, -34.75) (-53.825, -130.25, -34.75) (-53.825, -130.25, -5.25) (-68.425, -130.25, -5.25) on bodies 35 in component "edge-bracket_3d"